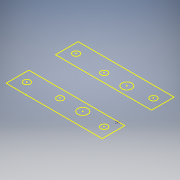
# Autodesk Inventor part: spool main support
Saved by Autodesk Inventor 2016 SP1 (Build 200210100, 210)
## iProperties
Created: 2016-04-23
Part Number: spool main support
Material: Generic
Document SubType Name: Modeling
Designer: ubik
Density: 1 g/cm^3
Appearance: Default
Author: ubik
Autodesk Inventor part; units mm, degrees
ref_plane "YZ Plane" through (0, 0, 0) normal (1, 0, 0) x (0, 1, 0)
ref_plane "XZ Plane" through (0, 0, 0) normal (0, 1, 0) x (-1, 0, 0)
ref_plane "XY Plane" through (0, 0, 0) normal (0, 0, 1) x (1, 0, 0)
sketch "Sketch1" plane through (0, 0, 0) normal (0, 0, 1) x (1, 0, 0)
  circle A0 centre (50, 45.5) radius 2.5 projected
  circle A1 centre (-8, 45.5) radius 2.5 projected
  circle A2 centre (32, 43.5) radius 3.75 projected
  circle A3 centre (15, 43.5) radius 2.4585 projected
  line L0 (57, 54) -> (-15, 54) projected
  line L1 (-15, 54) -> (-15, 37) projected
  line L2 (57, 37) -> (-15, 37) projected
  line L3 (57, 54) -> (57, 37) projected
  circle A4 centre (50, 8.5) radius 2.5 projected
  circle A5 centre (-8, 8.5) radius 2.5 projected
  circle A6 centre (32, 10.5) radius 3.75 projected
  circle A7 centre (15, 10.5) radius 2.4585 projected
  line L4 (57, 0) -> (-15, 0) projected
  line L5 (57, 0) -> (57, 17) projected
  line L6 (57, 17) -> (-15, 17) projected
  line L7 (-15, 0) -> (-15, 17) projected
  line L8 (-15, 107) -> (85, 107)
  line L9 (85, 107) -> (85, -53)
  line L10 (85, -53) -> (-15, -53)
  line L11 (-15, -53) -> (-15, 107)
  line L12 (-94.8305, 27) -> (141.7075, 27) construction
  circle A8 centre (-9, 27) radius 2.5
  circle A9 centre (79, 27) radius 2.5
  point P0 (0, 0)
  point P1 (52.2653, 16.3)
  dimension "d0" = 100
  dimension "d1" = 160
  dimension "d2" = 20
  dimension "d3" = 10
  dimension "d4" = 72
  dimension "d5" = 0
  dimension "d6" = 80
  dimension "d7" = 5
  dimension "d8" = 5
  dimension "d9" = 6
  dimension "d10" = 6
  constraints: 10 end point, 2 centre point, 2 horizontal, 2 parallel, 2 point on line, 1 perpendicular, 1 other
  measures "d0" distance between parallel lines of L9 L11
  measures "d1" distance of L10.end L8.start
  measures "d2" distance between parallel lines of L6 L2
  measures "d3" distance between parallel lines of L12 L2
  measures "d4" distance of L0.start L0.end
  measures "d5" distance between parallel lines of L11 L1
  measures "d6" distance between parallel lines of L12 L8
  measures "d7" diameter of A8
  measures "d8" diameter of A9
  measures "d9" distance from line of L11 A8.centre
  measures "d10" distance from line of L9 A9.centre
extrude "Extrusion1" add sketch "Sketch1" along normal blind 8
equation "\"d3\" = 0.5 * d2"
equation "\"d6\" = 0.5 * d1"
body "Solid1"
